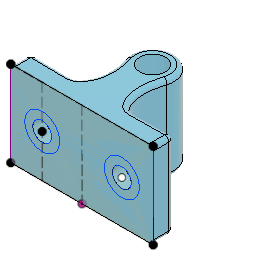
Z Lead Screw Restraint v3 (Autodesk Fusion 360 design; units mm, degrees)
Autodesk Fusion 360 part; units mm, degrees
sketch "Sketch1" plane through (0, 0, 0) normal (0, 1, 0) x (1, 0, 0) in component "Z Lead Screw"
  line L0 (0, 0) -> (0, -24.8) construction
  line L1 (0, -24.8) -> (-25, -24.8)
  line L2 (-25, -24.8) -> (-25, -17.8)
  line L3 (25, -24.8) -> (25, -17.8)
  line L4 (0, -24.8) -> (25, -24.8)
  spline S0 degree 5 poles (-25, -17.8) (-24.2148, -17.8) (-22.6415, -17.8016) (-20.2737, -17.8089) (-17.1801, -17.8376) (-13.837, -17.9297) (-11.3308, -18.0134) (-9.8302, -17.9312) (-8.6303, -17.213) (-7.251, -15.4367) (-6.0806, -12.4417) (-5.7762, -9.0008) (-6.1899, -5.8246) (-6.7922, -3.4416) (-7.175, -2.1838) knots 0 0 0 0 0 0 0.1 0.2 0.3 0.4 0.5 0.6 0.7 0.8 0.9 1 1 1 1 1 1
  line L5 (-30, -17.8) -> (-20, -17.8)
  line L6 (-11.5467, -18.2316) -> (-8.4533, -17.3684)
  spline S1 degree 5 poles (25, -17.8) (24.2148, -17.8) (22.6415, -17.8016) (20.2737, -17.8089) (17.1801, -17.8376) (13.837, -17.9297) (11.3308, -18.0134) (9.8302, -17.9312) (8.6303, -17.213) (7.251, -15.4367) (6.0806, -12.4417) (5.7762, -9.0008) (6.1899, -5.8246) (6.7922, -3.4416) (7.175, -2.1838) knots 0 0 0 0 0 0 0.1 0.2 0.3 0.4 0.5 0.6 0.7 0.8 0.9 1 1 1 1 1 1
  line L7 (-4.9333, -9.5491) -> (-9.4168, 5.1814)
  line L8 (30, -17.8) -> (20, -17.8)
  line L9 (11.5467, -18.2316) -> (8.4533, -17.3684)
  line L10 (4.9333, -9.5491) -> (9.4168, 5.1814)
  arc A0 (-7.175, -2.1838) -> (7.175, -2.1838) centre (0, 0) ccw construction
  line L11 (0, 0) -> (0, -4)
  arc A1 (7.175, -2.1838) -> (-7.175, -2.1838) centre (0, 0) ccw
  circle A2 centre (0, 0) radius 4.5
  dimension "d1" = 9
  dimension "d2" = 15
  dimension "d3" = 24.8
  dimension "d4" = 25
  dimension "d5" = 15
  dimension "d6" = 7
  dimension "d9" = 4
  measures "d1" diameter of A2
  measures "d2" diameter of A0
  measures "d6" distance of L0.start
  measures "d9" distance of L0.start
extrude "Extrude1" add sketch "Sketch1" along normal blind 30 in component "Z Lead Screw"
sketch "Sketch2" plane through (0, 0, 24.8) normal (0, 0, 1) x (1, 0, 0) in component "Z Lead Screw"
  line L0 (-25, 0) -> (25, 0)
  line L1 (25, 0) -> (25, 30)
  line L2 (25, 30) -> (-25, 30)
  line L3 (-25, 30) -> (-25, 0)
  line L4 (-25, 0) -> (-25, 30)
  line L5 (25, 0) -> (25, 30)
  line L6 (-25, 30) -> (25, 30) construction
  line L7 (25, 0) -> (-25, 0) construction
  line L8 (-25, 30) -> (-20, 30) construction
  line L9 (-20, 30) -> (-14, 30) construction
  line L10 (-14, 30) -> (-14, 0) construction
  circle A0 centre (-14, 15) radius 3.3
  circle A1 centre (-14, 15) radius 6.1
  line L11 (0, 30) -> (0, 0) construction
  circle A2 centre (14, 15) radius 6.1
  circle A3 centre (14, 15) radius 3.3
  dimension "d12" = 6
  dimension "d13" = 5
  measures "d12" distance of L11.end
extrude "Extrude2" cut sketch "Sketch2" against normal through all contours A0 | A3 in component "Z Lead Screw"
extrude "Extrude3" cut sketch "Sketch2" against normal blind 14 from surface at -4.5 contours A1 | A2 in component "Z Lead Screw"
fillet "Fillet1" radius 1.5 14 edges at (-9.08, 18.606, 17.3614) (20.0826, 15.4601, 17.8164) (9.9072, 30, 17.7726) (0, 30, -7.5) (-9.9072, 30, 17.7726) (-9.9072, 0, 17.7726) (9.9072, 0, 17.7726) (0, 0, -7.5) (25, 0, 21.3) (25, 15, 17.8) (25, 30, 21.3) (-25, 30, 21.3) (-25, 15, 17.8) (-25, 0, 21.3) in component "Z Lead Screw"
component "Z Lead Screw" placed x (1, 0, 0) y (0, 1, 0) z (0, 0, 1) at (0, 0, 0)
equation "d2 = d1 + 6 mm"
